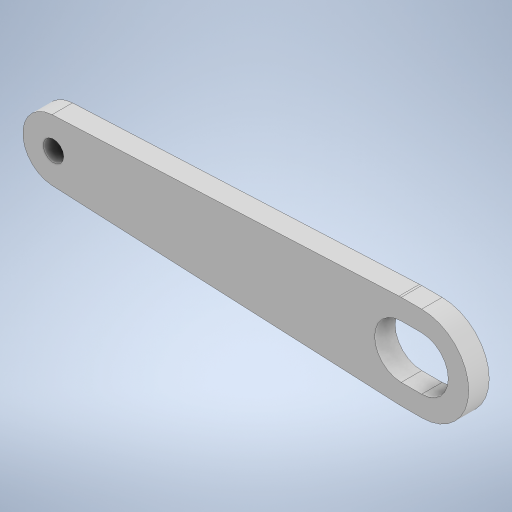
# Autodesk Inventor part: rotasyonpini
Saved by Autodesk Inventor 2023.2 (Build 272271000, 271)
## iProperties
Created: 2022-11-27
Part Number: rotasyonpini
Material: Generic
Document SubType Name: Modeling
Designer: omrfrkmll
Density: 1 g/cm^3
Appearance: Default
Author: omrfrkmll
Autodesk Inventor part; units mm, degrees
ref_plane "YZ Plane" through (0, 0, 0) normal (1, 0, 0) x (0, 1, 0)
ref_plane "XZ Plane" through (0, 0, 0) normal (0, 1, 0) x (-1, 0, 0)
ref_plane "XY Plane" through (0, 0, 0) normal (0, 0, 1) x (1, 0, 0)
sketch "Sketch1" plane through (0, 0, 0) normal (0, 0, 1) x (1, 0, 0)
  circle A0 centre (0, 0) radius 1
  arc A1 (34, 2.6) -> (34, -2.6) centre (34, 0) ccw
  line L0 (34, 2.6) -> (36, 2.6)
  line L1 (34, -2.6) -> (36, -2.6)
  arc A2 (36, -2.6) -> (36, 2.6) centre (36, 0) ccw
  arc A3 (-0.1412, 2.9967) -> (-0.1412, -2.9967) centre (0, 0) ccw
  line L2 (34, 4.6) -> (36, 4.6)
  arc A4 (36, -4.6) -> (36, 4.6) centre (36, 0) ccw
  line L3 (36, -4.6) -> (34, -4.6)
  line L4 (-0.1412, 2.9967) -> (33.7835, 4.5949)
  line L5 (12.7162, 0) -> (28.1806, 0)
  line L6 (-0.1412, -2.9967) -> (33.7835, -4.5949)
  arc A5 (34, 4.6) -> (33.7835, 4.5949) centre (34, 0) ccw
  arc A6 (33.7835, -4.5949) -> (34, -4.6) centre (34, 0) ccw
  dimension "d0" = 2
  dimension "d1" = 5.2
  dimension "d2" = 34
  dimension "d3" = 2
  dimension "d4" = 2
  constraints: 14 end point, 12 point on circle, 7 centre point, 4 horizontal, 4 tangent, 2 symmetric about line, 1 coincident, 2 other
  measures "d0" diameter of A0
  measures "d1" diameter of A1
  measures "d2" distance of A1.centre point (0, 0)
  measures "d3" distance of A2.centre A1.centre
  measures "d4" radial gap between concentric circles of A0 A3
extrude "Extrusion1" add sketch "Sketch1" along normal blind 2
body "Solid1"
